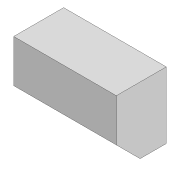
# Autodesk Inventor part: KR500 0.25 Model Stand
Saved by Autodesk Inventor 2020 (Build 240168000, 168)
## iProperties
Created: 2021-07-01
Part Number: KR500 0.25 Model Stand
Material: Generic
Document SubType Name: Modeling
Designer: Coy
Density: 1 g/cm^3
Appearance: Default
Author: Coy
Autodesk Inventor part; units mm, degrees
ref_plane "YZ Plane" through (0, 0, 0) normal (1, 0, 0) x (0, 1, 0)
ref_plane "XZ Plane" through (0, 0, 0) normal (0, 1, 0) x (-1, 0, 0)
ref_plane "XY Plane" through (0, 0, 0) normal (0, 0, 1) x (1, 0, 0)
sketch "Sketch1" plane through (0, 0, 0) normal (0, 0, 1) x (1, 0, 0)
  line L0 (21.4889, 22.1562) -> (198.9889, 22.1562) construction
  line L1 (198.9889, 22.1562) -> (198.9889, 137.1562) construction
  line L2 (198.9889, 137.1562) -> (21.4889, 137.1562) construction
  line L3 (21.4889, 137.1562) -> (21.4889, 22.1562) construction
  line L4 (0, 0) -> (220, 0) construction
  line L5 (220, 0) -> (220, 220) construction
  line L6 (220, 220) -> (0, 220) construction
  line L7 (0, 220) -> (0, 0) construction
  line L8 (11.3161, 9.8062) -> (227.2161, 9.8062)
  line L9 (227.2161, 9.8062) -> (227.2161, 149.5062)
  line L10 (227.2161, 149.5062) -> (11.3161, 149.5062)
  line L11 (11.3161, 149.5062) -> (11.3161, 9.8062)
  line L12 (21.4889, 137.1562) -> (21.4889, 149.5062) construction
  line L13 (21.4889, 22.1562) -> (21.4889, 9.8062) construction
  line L14 (16.3161, 144.5062) -> (222.2161, 144.5062)
  line L15 (222.2161, 144.5062) -> (222.2161, 14.8062)
  line L16 (222.2161, 14.8062) -> (16.3161, 14.8062)
  line L17 (16.3161, 14.8062) -> (16.3161, 144.5062)
  dimension "d0" = 177.5
  dimension "d1" = 115
  dimension "d2" = 220
  dimension "d3" = 220
  dimension "d4" = 0
  dimension "d5" = 0
  dimension "d6" = 215.9
  dimension "d7" = 139.7
  dimension "d8" = 5
  constraints: 36 end point, 8 parallel, 5 perpendicular, 3 horizontal, 3 point on line, 1 collinear, 3 other
  measures "d0" distance of L2.end L1.end
  measures "d1" distance of L1.end L0.end
  measures "d2" distance of L6.end L5.end
  measures "d3" distance of L5.end L4.end
  measures "d4" distance of point (0, 0) L4.start
  measures "d5" distance of point (0, 0) L4.start
  measures "d6" distance of L10.end L9.end
  measures "d7" distance of L9.end L8.end
  measures "d8" distance between parallel lines of L10 L14
extrude "Extrusion1" add sketch "Sketch1" along normal blind 5 contours L11 L10 L9 L8 | L14 L15 L16 L17
sketch "Sketch2" plane through (0, 0, 5) normal (0, 0, 1) x (1, 0, 0)
  line L0 (227.2161, 149.5062) -> (11.3161, 149.5062) projected
  line L1 (11.3161, 149.5062) -> (11.3161, 9.8062) projected
  line L2 (11.3161, 9.8062) -> (227.2161, 9.8062) projected
  line L3 (227.2161, 9.8062) -> (227.2161, 149.5062) projected
  line L4 (16.3161, 14.8062) -> (16.3161, 144.5062)
  line L5 (16.3161, 144.5062) -> (222.2161, 144.5062)
  line L6 (222.2161, 144.5062) -> (222.2161, 14.8062)
  line L7 (222.2161, 14.8062) -> (16.3161, 14.8062)
  point P0 (0, 0)
  dimension "d11" = 5
  constraints: 8 end point, 3 other
  measures "d11" distance between parallel lines of L1 L4
extrude "Extrusion2" add sketch "Sketch2" along normal blind 50
sketch "Sketch3" plane through (11.3161, 9.8062, 0) normal (-1, 0, 0) x (0, 0, 1)
  line L0 (0, 139.7) -> (55, 139.7) projected
  line L1 (55, 139.7) -> (105, 139.7)
  line L2 (55, 0) -> (105, 50)
  line L3 (55, 139.7) -> (55, 0) projected
  line L4 (105, 139.7) -> (105, 50)
  point P0 (0, -9.8062)
  dimension "d14" = 50
  dimension "d15" = 45
  constraints: 6 end point, 1 horizontal, 1 vertical
  measures "d14" distance of L0.end L1.end
  measures "d15" angle of L3 L2
extrude "Extrusion3" add sketch "Sketch3" against normal blind 5
sketch "Sketch4" plane through (16.3161, 14.8062, 5) normal (1, 0, 0) x (0, 0, -1)
  line L0 (-100, 45) -> (-50, -5) projected
  line L1 (-100, 134.7) -> (-100, 45) projected
  line L2 (-50, 134.7) -> (-100, 134.7) projected
  line L3 (-46.4645, -1.4645) -> (-95, 47.0711)
  line L4 (-95, 47.0711) -> (-95, 129.7)
  line L5 (-95, 129.7) -> (-50, 129.7)
  line L6 (-50, 134.7) -> (-50, 129.7) projected
  line L7 (0, 129.7) -> (0, 0) projected
  line L8 (0, 129.7) -> (-50, 129.7) projected
  line L9 (-50, 134.7) -> (-50, 129.7) projected
  line L10 (-50, 134.7) -> (-100, 134.7) projected
  line L11 (-100, 134.7) -> (-100, 45) projected
  line L12 (-100, 45) -> (-50, -5) projected
  line L13 (-50, 0) -> (-50, -5) projected
  line L14 (0, 0) -> (-50, 0) projected
  point P0 (5, -14.8062)
  point P1 (-50, -5)
  point P2 (-47.9289, 0)
  dimension "d18" = 5
  constraints: 6 end point, 2 other
  measures "d18" distance between parallel lines of L0 L3
extrude "Extrusion4" add sketch "Sketch4" along normal up to surface (205.9 mm away) contours L1 L2 L6 L5 L4 L3 L14 L13 L0
sketch "Sketch5" plane through (222.2161, 59.8062, 105) normal (1, 0, 0) x (0, 0, -1)
  line L0 (50, -42.9289) -> (50, -50) projected
  line L1 (50, -42.9289) -> (5, 2.0711) projected
  line L2 (5, 2.0711) -> (5, 84.7) projected
  line L3 (5, 84.7) -> (50, 84.7) projected
  line L4 (50, 89.7) -> (50, 84.7) projected
  line L5 (50, 89.7) -> (0, 89.7) projected
  line L6 (0, 89.7) -> (0, 0) projected
  line L7 (0, 0) -> (50, -50) projected
  line L8 (50, 84.7) -> (50, -42.9289) projected
  point P0 (105, -59.8062)
extrude "Extrusion5" add sketch "Sketch5" along normal blind 5
body "Solid1"
